board v2 (Autodesk Fusion 360 design; units mm, degrees)
Autodesk Fusion 360 part; units mm, degrees
sketch "スケッチ1" plane through (0, 0, 0) normal (0, 0, 1) x (1, 0, 0)
  line L0 (0, 0) -> (-12.5, 0)
  line L1 (-12.5, 0) -> (-12.5, 12)
  line L2 (-12.5, 12) -> (0, 12)
  line L3 (0, 12) -> (0, 0)
  line L4 (0, 0) -> (12.5, 0)
  line L5 (12.5, 0) -> (12.5, 12)
  line L6 (12.5, 12) -> (0, 12)
  line L7 (0, 12) -> (0, 0)
  line L8 (0, 0) -> (-12.5, 0)
  line L9 (-12.5, 0) -> (-12.5, -10.5)
  line L10 (-12.5, -10.5) -> (0, -10.5)
  line L11 (0, -10.5) -> (0, 0)
  line L12 (0, 0) -> (12.5, 0)
  line L13 (12.5, 0) -> (12.5, -10.5)
  line L14 (12.5, -10.5) -> (0, -10.5)
  line L15 (0, -10.5) -> (0, 0)
  line L16 (0, -10.5) -> (-9, -10.5)
  line L17 (-9, -10.5) -> (-9, -13)
  line L18 (-9, -13) -> (0, -13)
  line L19 (0, -13) -> (0, -10.5)
  line L20 (0, -10.5) -> (9, -10.5)
  line L21 (9, -10.5) -> (9, -13)
  line L22 (9, -13) -> (0, -13)
  line L23 (0, -13) -> (0, -10.5)
  line L24 (-12.5, 12) -> (-18.5, 12)
  line L25 (12.5, 12) -> (18.5, 12)
  arc A0 (-2.5, 28) -> (-18.5, 12) centre (-2.5, 12) ccw
  arc A1 (18.5, 12) -> (2.5, 28) centre (2.5, 12) ccw
  line L26 (-2.5, 28) -> (2.5, 28)
  circle A2 centre (-11, 7) radius 0.8
  circle A3 centre (-11, -7) radius 0.8
  circle A4 centre (11, -7) radius 0.8
  circle A5 centre (11, 7) radius 0.8
  circle A6 centre (0, 10.5) radius 6
  line L27 (0, 12) -> (0, 28)
  dimension "d1" = 6
  dimension "d2" = 12.5
  dimension "d3" = 12
  dimension "d4" = 28
  dimension "d5" = 1.6
  dimension "d6" = 7
  dimension "d7" = 3.5
  dimension "d8" = 3.5
  dimension "d9" = 2.5
  dimension "d10" = 12
  dimension "d11" = 10.5
  dimension "d17" = 22
  measures "d1" distance of L1.end L24.end
  measures "d2" distance of L9.end L10.end
  measures "d3" distance of L0.end L1.end
  measures "d4" distance of L12 L26
  measures "d5" diameter of A2
  measures "d6" distance of L0 A2.centre
  measures "d7" distance of L10 A3.centre
  measures "d8" distance of L9.end L16.end
  measures "d9" distance of L16.end L17.end
  measures "d10" diameter of A6
  measures "d11" distance of L0.start A6.centre
  measures "d17" distance of A3.centre A4.centre
extrude "押し出し1" add sketch "スケッチ1" along normal blind 0.6 contours L0 L8 L9 L10 L11 L15 L16 | L0 L1 L2 L3 L7 L8 A6 | L3 L4 L5 L6 L7 L12 A6 | L4 L11 L12 L13 L14 L15 L20 | L10 L16 L17 L18 L19 L23 | L14 L19 L20 L21 L22 L23 | L2 L24 A0 L26 A6 L27 | L6 L25 A1 L26 A6 L27
fillet "フィレット1" radius 3 2 edges at (-18.5, 12, 0.3) (18.5, 12, 0.3)
fillet "フィレット1" radius 2 2 edges at (-12.5, 12, 0.3) (12.5, 12, 0.3)
fillet "フィレット1" radius 1 6 edges at (-12.5, -10.5, 0.3) (-9, -10.5, 0.3) (-9, -13, 0.3) (9, -13, 0.3) (9, -10.5, 0.3) (12.5, -10.5, 0.3)
